led_lead_cutting_guide (Autodesk Fusion 360 design; units mm, degrees)
Autodesk Fusion 360 part; units mm, degrees
note: some values were not read from the file. Chosen so that the rebuilt part matches the saved one: which face or edge a step refers to.
sketch "Sketch2" plane through (0, 0, 0) normal (0, 0, 1) x (1, 0, 0)
  circle A0 centre (0, 0) radius 1.55
  line L0 (-1.55, 1.3416) -> (-1.55, -1.3416)
  arc A1 (-1.55, -1.3416) -> (-1.55, 1.3416) centre (0, 0) ccw
  dimension "d26" = 3.1
  dimension "d27" = 4.1
  dimension "d37" = 0
  dimension "d38" = 0
  dimension "d39" = 0
  dimension "d40" = 0
  dimension "d49" = 0
  dimension "d50" = 0
  dimension "d51" = 0
  dimension "d52" = 0
  measures "d26" diameter of A0
  measures "d27" diameter of A1
extrude "Extrude1" add sketch "Sketch2" along normal blind 3.2 contours A0 makes body 1
extrude "Extrude2" add sketch "Sketch2" against normal blind 0.75 contours A0 | L0 A1 bodies 1
sketch "Sketch3" plane through (0, 0, -0.75) normal (0, 0, -1) x (1, 0, 0)
  arc A0 (-1.55, -1.3416) -> (-1.55, 1.3416) centre (0, 0) ccw
  line L0 (-1.55, 1.3416) -> (-1.55, -1.3416)
  line L1 (-1.55, 0) -> (2.05, 0) construction
  line L2 (-1.55, 0.25) -> (-1.05, 0.25)
  line L3 (-1.05, 0.25) -> (-1.05, -0.25)
  line L4 (-1.05, -0.25) -> (-1.55, -0.25)
  line L5 (-1.55, -0.25) -> (-1.55, 0.25)
  line L6 (0.99, 0.25) -> (1.49, 0.25)
  line L7 (1.49, 0.25) -> (1.49, -0.25)
  line L8 (1.49, -0.25) -> (0.99, -0.25)
  line L9 (0.99, -0.25) -> (0.99, 0.25)
  line L10 (-1.3, -0.25) -> (-1.3, 0.25) construction
  line L11 (1.24, -0.25) -> (1.24, 0.25) construction
  point P0 (-1.55, 0)
  dimension "d32" = 2.54
  dimension "d33" = 0.5
  dimension "d34" = 0.5
  measures "d32" distance of L10 L11
  measures "d33" distance of L2.end L3.end
  measures "d34" distance of L2.start L2.end
extrude "Extrude3" add sketch "Sketch3" along normal blind 4.4 contours L0 L2 L3 L4 L5 | L6 L7 L8 L9 bodies 1
sketch "Sketch1" plane through (0, 0, -0.75) normal (0, 0, -1) x (1, 0, 0) in component "Component"
  line L0 (0.99, -0.25) -> (0.99, 0.25)
  line L1 (0.99, 0.25) -> (1.49, 0.25)
  line L2 (1.49, 0.25) -> (1.49, -0.25)
  line L3 (1.49, -0.25) -> (0.99, -0.25)
  line L4 (-1.55, 0.25) -> (-1.05, 0.25)
  line L5 (-1.05, 0.25) -> (-1.05, -0.25)
  line L6 (-1.05, -0.25) -> (-1.55, -0.25)
  line L7 (-1.55, -0.25) -> (-1.55, -1.3416)
  arc A0 (-1.55, -1.3416) -> (-1.55, 1.3416) centre (0, 0) ccw
  line L8 (-1.55, 1.3416) -> (-1.55, 0.25)
  circle A1 centre (0, 0) radius 3
  line L9 (0.99, 0) -> (1.49, 0) construction
  line L10 (1.24, 0.25) -> (1.24, -0.25) construction
  line L11 (-1.3, 0.25) -> (-1.3, -0.25) construction
  line L12 (-1.05, 0) -> (-1.55, 0) construction
  circle A2 centre (-1.3, 0) radius 1
  circle A3 centre (1.24, 0) radius 1
  point P0 (-1.55, 0)
  dimension "d1" = 6
  dimension "d2" = 2
  measures "d1" diameter of A1
  measures "d2" diameter of A3
extrude "Extrude1'" add sketch "Sketch1" along normal up to surface (4.4 mm away) separate body contours L7 A0 L8 A2 A3 | A1 makes body 2 in component "Component"
sketch "Sketch2 (2)" plane through (0, 0, -5.15) normal (0, 0, -1) x (1, 0, 0) in component "Component"
  circle A0 centre (0, 0) radius 3
  circle A1 centre (-1.3, 0) radius 1
  circle A2 centre (1.24, 0) radius 1
  line L0 (-23, 2.5) -> (23, 2.5)
  line L1 (23, 2.5) -> (23, -2.5)
  line L2 (23, -2.5) -> (-23, -2.5)
  line L3 (-23, -2.5) -> (-23, 2.5)
  line L4 (23, 0) -> (-23, 0) construction
  line L5 (0, 2.5) -> (0, -2.5) construction
  dimension "d6" = 20
  dimension "d7" = 5
  measures "d6" distance of A0 L1
  measures "d7" distance of L0.start L2.end
extrude "Extrude2'" add sketch "Sketch2 (2)" against normal blind 3 contours A0 L0 L1 L2 | A0 L0 L2 L3 bodies 2 in component "Component"
fillet "Fillet1" radius 2 4 edges at (23, -2.5, -3.65) (23, 2.5, -3.65) (-23, -2.5, -3.65) (-23, 2.5, -3.65) on bodies 2 in component "Component"
fillet "Fillet2" radius 1.5 10 edges at (-11.3292, 2.5, -2.15) (-22.4142, 1.9142, -2.15) (-23, 0, -2.15) (-22.4142, -1.9142, -2.15) (-11.3292, -2.5, -2.15) (11.3292, -2.5, -2.15) (22.4142, -1.9142, -2.15) (23, 0, -2.15) (22.4142, 1.9142, -2.15) (11.3292, 2.5, -2.15) on bodies 2 in component "Component"
fillet "Fillet3" radius 0.5 1 edges at (-2.797, 1.0848, -0.75) on bodies 2 in component "Component"
component "Component" placed x (1, 0, 0) y (0, 1, 0) z (0, 0, 1) at (0, 0, 0)
